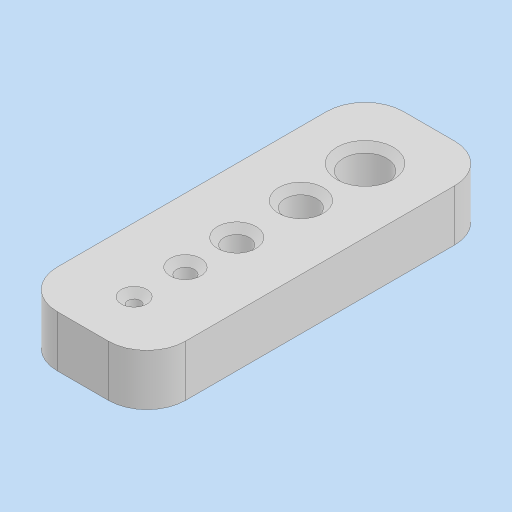
# Autodesk Inventor part: hole_size_test
Saved by Autodesk Inventor 2024 (Build 280153000, 153)
## iProperties
Created: 2025-05-12
Part Number: hole_size_test
Material: Generic
Document SubType Name: Modeling
Designer: XxPan
Density: 1 g/cm^3
Appearance: Default
Author: XxPan
Autodesk Inventor part; units mm, degrees
ref_plane "YZ Plane" through (0, 0, 0) normal (1, 0, 0) x (0, 1, 0)
ref_plane "XZ Plane" through (0, 0, 0) normal (0, 1, 0) x (-1, 0, 0)
ref_plane "XY Plane" through (0, 0, 0) normal (0, 0, 1) x (1, 0, 0)
sketch "Sketch1" plane through (0, 0, 0) normal (0, 1, 0) x (-1, 0, 0)
  circle A0 centre (0, 0) radius 1
  circle A1 centre (0, 4) radius 0.7
  circle A2 centre (0, -10) radius 1.7
  circle A3 centre (0, 8) radius 0.5
  circle A4 centre (0, -5) radius 1.25
  line L0 (5, 12) -> (-5, 12)
  line L1 (-5, 12) -> (-5, -15)
  line L2 (-5, -15) -> (5, -15)
  line L3 (5, -15) -> (5, 12)
  dimension "d0" = 2
  dimension "d1" = 1.4
  dimension "d2" = 3.4
  dimension "d3" = 1
  dimension "d4" = 2.5
  dimension "d5" = 4
  dimension "d6" = 4
  dimension "d7" = 5
  dimension "d8" = 5
  dimension "d11" = 4
  dimension "d12" = 5
  dimension "d13" = 5
  dimension "d14" = 5
  constraints: 8 end point, 5 centre point, 2 parallel, 1 coincident, 1 horizontal, 1 perpendicular
  measures "d0" diameter of A0
  measures "d1" diameter of A1
  measures "d2" diameter of A2
  measures "d3" diameter of A3
  measures "d4" diameter of A4
  measures "d5" distance of A1.centre A3.centre
  measures "d6" distance of point (0, 0) A1.centre
  measures "d7" distance of A4.centre point (0, 0)
  measures "d8" distance of A2.centre A4.centre
  measures "d11" distance from line of L0 A3.centre
  measures "d12" distance from line of A2.centre L2
  measures "d13" distance from line of L3 A2.centre
  measures "d14" distance from line of L1 A2.centre
extrude "Extrusion1" add sketch "Sketch1" along normal blind 4
fillet "Fillet1" radius 3 4 edges at (5, 2, 12) (-5, 2, 12) (-5, 2, -15) (5, 2, -15)
chamfer "Chamfer1" distance 0.5 angle 45 5 edges at (1.7, 4, -10) (1.25, 4, -5) (1, 4, 0) (0.7, 4, 4) (0.5, 4, 8)
body "Solid1"
